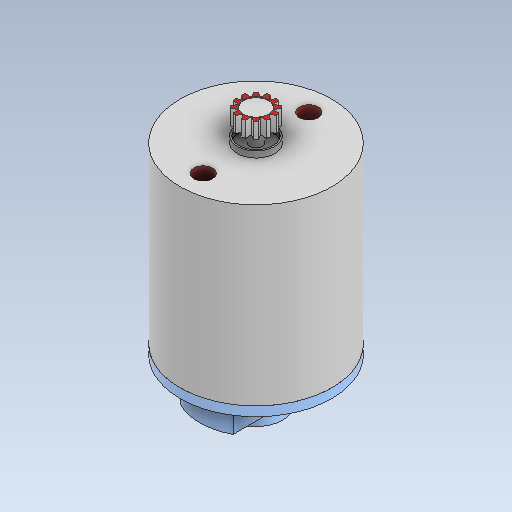
# Autodesk Inventor part: MOTOR_DETAL
Saved by Autodesk Inventor 2020 (Build 240168000, 168)
## iProperties
Created: 2019-10-21
Part Number: MOTOR_DETAL
Material: Ogólny
Document SubType Name: Modeling
Designer: atmat
Density: 1 g/cm^3
Appearance: Domyślna
Author: atmat
Autodesk Inventor part; units mm, degrees
ref_plane "YZ Plane" through (0, 0, 0) normal (1, 0, 0) x (0, 1, 0)
ref_plane "XZ Plane" through (0, 0, 0) normal (0, 1, 0) x (-1, 0, 0)
ref_plane "XY Plane" through (0, 0, 0) normal (0, 0, 1) x (1, 0, 0)
sketch "Szkic1" plane through (0, 0, 0) normal (0, 1, 0) x (-1, 0, 0)
  circle A0 centre (0, 0) radius 12.2
  dimension "d0" = 24.4
  constraints: 1 centre point, 1 coincident
  measures "d0" diameter of A0
extrude "Wyciągnięcie proste1" add sketch "Szkic1" along normal blind 28
sketch "Szkic2" plane through (0, 28, 0) normal (0, 1, 0) x (1, 0, 0)
  circle A0 centre (0, 0) radius 3
  dimension "d3" = 6
  constraints: 1 centre point, 1 coincident
  measures "d3" diameter of A0
extrude "Wyciągnięcie proste2" add sketch "Szkic2" along normal blind 1
sketch "Szkic3" plane through (0, 29, 0) normal (0, 1, 0) x (1, 0, 0)
  circle A0 centre (0, 0) radius 2.75
  dimension "d6" = 5.5
  constraints: 1 centre point, 1 coincident
  measures "d6" diameter of A0
extrude "Wyciągnięcie proste3" cut sketch "Szkic3" against normal blind 1
sketch "Szkic4" plane through (0, 28, 0) normal (0, 1, 0) x (1, 0, 0)
  circle A0 centre (0, 0) radius 1
  dimension "d9" = 2
  constraints: 1 centre point, 1 coincident
  measures "d9" diameter of A0
extrude "Wyciągnięcie proste4" add sketch "Szkic4" along normal blind 5
sketch "Szkic5" plane through (0, 33, 0) normal (0, 1, 0) x (1, 0, 0)
  circle A0 centre (0, 0) radius 2.875
  dimension "d12" = 5.75
  constraints: 1 centre point, 1 coincident
  measures "d12" diameter of A0
extrude "Wyciągnięcie proste5" add sketch "Szkic5" against normal blind 2.5
sketch "Szkic6" plane through (0, 33, 0) normal (0, 1, 0) x (1, 0, 0)
  circle A0 centre (0, 0) radius 2
  line L0 (0, 2) -> (-0.4817, 2.8344)
  circle A1 centre (0, 0) radius 2.875 projected
  line L1 (0, 2) -> (0, 2.875) construction
  line L2 (0, 2) -> (0.4817, 2.8344)
  arc A2 (0.4817, 2.8344) -> (-0.4817, 2.8344) centre (0, 0) ccw
  dimension "d15" = 4
  dimension "d16" = 30
  dimension "d24" = 30
  constraints: 6 end point, 6 point on circle, 1 centre point, 1 coincident, 1 vertical, 1 vertical alignment, 2 other
  measures "d16" angle of L1 L0
  measures "d24" angle of L1 L2
extrude "Wyciągnięcie proste6" cut sketch "Szkic6" against normal blind 2.5 contours L0 A1 L2 picked at (0.2143, 2.5683)
sketch "Szkic7" plane through (0, 33, 0) normal (0, 1, 0) x (1, 0, 0)
  line L0 (-0.4817, 2.8344) -> (0, 2) projected
  circle A0 centre (0, 0) radius 2
  constraints: 1 coincident, 1 vertical alignment, 2 other
extrude "Wyciągnięcie proste7" cut sketch "Szkic7" against normal blind 0.1
pattern_circular "Szyk kołowy1" count 12 over 360 about axis through (0, -10, 0) along (0, 1, 0) of "Wyciągnięcie proste6"
sketch "Szkic8" plane through (0, 28, 0) normal (0, 1, 0) x (1, 0, 0)
  circle A0 centre (0, -8.5) radius 1.5
  circle A1 centre (0, 8.5) radius 1.5
  point P0 (0, 0)
  dimension "d25" = 3
  dimension "d26" = 3
  dimension "d27" = 17
  dimension "d28" = 8.5
  constraints: 2 centre point
  measures "d25" diameter of A0
  measures "d26" diameter of A1
  measures "d27" distance of A1.centre A0.centre
  measures "d28" distance of point (0, 0) A0.centre
extrude "Wyciągnięcie proste8" cut sketch "Szkic8" against normal blind 2
sketch "Szkic9" plane through (0, 0, 0) normal (0, -1, 0) x (1, 0, 0)
  circle A0 centre (0, 0) radius 12.2
  dimension "d41" = 24.4
  constraints: 1 centre point, 1 coincident
  measures "d41" diameter of A0
extrude "Wyciągnięcie proste9" add sketch "Szkic9" along normal blind 1.5 separate body
sketch "Szkic10" plane through (0, -1.5, 0) normal (0, -1, 0) x (1, 0, 0)
  line L0 (-4.25, -7.9333) -> (4.25, -7.9333)
  line L1 (4.25, -7.9333) -> (4.25, 7.9333)
  line L2 (4.25, 7.9333) -> (-4.25, 7.9333)
  line L3 (-4.25, 7.9333) -> (-4.25, -7.9333)
  circle A0 centre (0, 0) radius 9
  point P0 (4.25, -7.9333)
  dimension "d33" = 8.5
  dimension "d34" = 4.25
  dimension "d35" = 18
  constraints: 8 end point, 2 parallel, 2 point on circle, 1 centre point, 1 coincident, 1 horizontal, 1 perpendicular
  measures "d33" distance of L1.end L2.end
  measures "d34" distance from line of point (0, 0) L3
  measures "d35" diameter of A0
extrude "Wyciągnięcie proste10" add sketch "Szkic10" along normal blind 5 contours L3 L2 L1 L0 | L0 A0 | A0 L2 bodies 2
sketch "Szkic11" plane through (0, -6.5, 0) normal (0, -1, 0) x (1, 0, 0)
  circle A0 centre (0, 0) radius 4.25
  dimension "d38" = 8.5
  constraints: 1 centre point, 1 coincident
  measures "d38" diameter of A0
extrude "Wyciągnięcie proste11" add sketch "Szkic11" along normal blind 2 bodies 2
